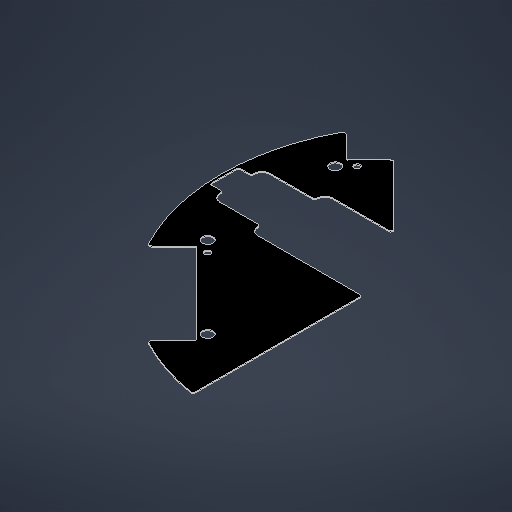
# Autodesk Inventor part: Cover Left
Saved by Autodesk Inventor 2026.1 (Build 301233020, 233B)
## iProperties
Created: 2026-06-25
Part Number: Cover Left
Material: Generic
Document SubType Name: Modeling
Designer: Bahaa
Mass: 3.13379 g
Surface Area: 128.68 cm^2
Volume: 3.13379 cm^3
Density: 1 g/cm^3
Appearance: Black PLA
Author: Bahaa
Autodesk Inventor part; units mm, degrees
ref_plane "YZ Plane" through (0, 0, 0) normal (1, 0, 0) x (0, 1, 0)
ref_plane "XZ Plane" through (0, 0, 0) normal (0, 1, 0) x (-1, 0, 0)
ref_plane "Work Plane1" through (0, 0, 0) normal (0, 0, 1) x (1, 0, 0)
sketch "Sketch1" plane through (0, 0, 0) normal (0, 0, 1) x (1, 0, 0)
  line L0 (-6.390879, 14.118801) -> (-6.390879, 24.738784)
  arc A0 (-4.409747, 26.159527) -> (-6.390879, 24.738784) centre (-4.890879, 24.738784) ccw
  arc A1 (11.10009, 19.508657) -> (-4.409747, 26.159527) centre (-38.890879, -75.660419) ccw
  arc A2 (11.463202, 17.120056) -> (11.10009, 19.508657) centre (10.402541, 18.180716) ccw
  line L1 (11.463202, 17.120056) -> (0.353553, 6.010408)
  arc A3 (-0.353553, 6.010408) -> (0.353553, 6.010408) centre (0, 6.363961) ccw
  line L2 (-0.353553, 6.010408) -> (-4.926413, 10.583267)
  arc A4 (-6.390879, 14.118801) -> (-4.926413, 10.583267) centre (-1.390879, 14.118801) ccw
  arc A5 (-78.135299, 6.01042) -> (-77.428193, 6.01042) centre (-77.781746, 6.363974) ccw
  line L3 (-78.135299, 6.01042) -> (-89.244944, 17.120065)
  arc A6 (-88.881832, 19.508666) -> (-89.244944, 17.120065) centre (-88.184283, 18.180725) ccw
  arc A7 (-73.372011, 26.159527) -> (-88.881832, 19.508666) centre (-38.890879, -75.660419) ccw
  arc A8 (-71.390879, 24.738784) -> (-73.372011, 26.159527) centre (-72.890879, 24.738784) ccw
  line L4 (-71.390879, 24.738784) -> (-71.390879, 14.118801)
  arc A9 (-72.855345, 10.583267) -> (-71.390879, 14.118801) centre (-76.390879, 14.118801) ccw
  line L5 (-72.855345, 10.583267) -> (-77.428193, 6.01042)
  circle A10 centre (-1.978787, -172.354511) radius 2.85
  circle A11 centre (36.76954, -114.551299) radius 1.6
  circle A12 centre (-114.551311, -114.551286) radius 1.6
  circle A13 centre (-114.551299, -36.76954) radius 1.6
  circle A14 centre (36.769553, -36.769553) radius 1.6
  circle A15 centre (-77.781759, -151.320838) radius 2.85
  circle A16 centre (-0.000013, -151.320851) radius 2.85
  circle A17 centre (42.426394, -108.894444) radius 2.85
  circle A18 centre (42.426394, -42.426394) radius 2.85
  circle A19 centre (-120.208153, -42.426394) radius 2.85
  circle A20 centre (-120.208153, -108.894444) radius 2.85
  arc A21 (-134.059964, -125.651371) -> (-131.671363, -126.014483) centre (-132.732023, -124.953823) ccw
  arc A22 (-134.059955, -25.66945) -> (-134.059964, -125.651371) centre (-38.890879, -75.660419) ccw
  arc A23 (-131.671354, -25.306338) -> (-134.059955, -25.66945) centre (-132.732015, -26.366998) ccw
  line L6 (-131.671354, -25.306338) -> (-120.561706, -36.415986)
  arc A24 (-120.561706, -36.415986) -> (-119.854599, -36.415986) centre (-120.208153, -36.062433) ccw
  line L7 (-119.854599, -36.415986) -> (-83.4386, 0.000013)
  line L8 (-83.4386, 0.000013) -> (-80.903066, -2.535521)
  arc A25 (-81.106225, -2.960902) -> (-80.903066, -2.535521) centre (-81.079843, -2.712298) ccw
  arc A26 (-81.106225, -2.960902) -> (-82.731493, -3.535521) centre (-81.31728, -4.949735) ccw
  line L9 (-82.731493, -3.535521) -> (-111.015777, -31.819805)
  arc A27 (-111.015777, -31.819805) -> (-111.015777, -34.648232) centre (-109.601564, -33.234019) ccw
  line L10 (-111.015777, -34.648232) -> (-110.308671, -35.355339)
  arc A28 (-110.308671, -38.183766) -> (-110.308671, -35.355339) centre (-111.722884, -36.769553) ccw
  line L11 (-110.308671, -38.183766) -> (-118.793939, -46.669035)
  arc A29 (-121.622366, -46.669035) -> (-118.793939, -46.669035) centre (-120.208153, -45.254821) ccw
  line L12 (-121.622366, -46.669035) -> (-128.634815, -39.656586)
  arc A30 (-128.634815, -39.656586) -> (-131.91894, -40.361269) centre (-130.049029, -41.0708) ccw
  arc A31 (-131.91894, -40.361269) -> (-138.034364, -67.24499) centre (-38.890879, -75.660419) ccw
  arc A32 (-139.030781, -68.160413) -> (-138.034364, -67.24499) centre (-139.030781, -67.160413) ccw
  line L13 (-139.030781, -68.160413) -> (-143.890873, -68.160413)
  arc A33 (-143.890873, -68.160413) -> (-144.890873, -69.160413) centre (-143.890873, -69.160413) ccw
  line L14 (-144.890873, -69.160413) -> (-144.890873, -82.160413)
  arc A34 (-144.890873, -82.160413) -> (-143.890873, -83.160413) centre (-143.890873, -82.160413) ccw
  line L15 (-143.890873, -83.160413) -> (-139.030782, -83.160413)
  arc A35 (-138.034365, -84.075836) -> (-139.030782, -83.160413) centre (-139.030782, -84.160413) ccw
  arc A36 (-138.034365, -84.075836) -> (-131.918947, -110.959551) centre (-38.890879, -75.660419) ccw
  arc A37 (-131.918947, -110.959551) -> (-128.634822, -111.664234) centre (-130.049036, -110.25002) ccw
  line L16 (-128.634822, -111.664234) -> (-121.622379, -104.651791)
  arc A38 (-118.793952, -104.651791) -> (-121.622379, -104.651791) centre (-120.208166, -106.066004) ccw
  line L17 (-118.793952, -104.651791) -> (-110.308671, -113.137072)
  arc A39 (-110.308671, -115.965499) -> (-110.308671, -113.137072) centre (-111.722884, -114.551286) ccw
  line L18 (-110.308671, -115.965499) -> (-111.015777, -116.672606)
  arc A40 (-111.015777, -116.672606) -> (-111.015777, -119.501033) centre (-109.601564, -118.08682) ccw
  line L19 (-111.015777, -119.501033) -> (-82.731493, -147.785317)
  arc A41 (-82.731493, -147.785317) -> (-79.903066, -147.785317) centre (-81.31728, -146.371104) ccw
  line L20 (-79.903066, -147.785317) -> (-79.195959, -147.07821)
  arc A42 (-76.367532, -147.07821) -> (-79.195959, -147.07821) centre (-77.781746, -148.492424) ccw
  line L21 (-76.367532, -147.07821) -> (-67.882264, -155.563479)
  arc A43 (-67.882264, -158.391906) -> (-67.882264, -155.563479) centre (-69.296477, -156.977693) ccw
  line L22 (-67.882264, -158.391906) -> (-74.894713, -165.404355)
  arc A44 (-74.894713, -165.404355) -> (-74.19003, -168.688479) centre (-73.480499, -166.818569) ccw
  arc A45 (-74.19003, -168.688479) -> (-56.419377, -173.60429) centre (-38.890879, -75.660419) ccw
  arc A46 (-56.419377, -173.60429) -> (-52.890879, -170.651208) centre (-55.890879, -170.651208) ccw
  line L23 (-52.890879, -170.651208) -> (-52.890879, -107.660419)
  arc A47 (-49.890879, -104.660419) -> (-52.890879, -107.660419) centre (-49.890879, -107.660419) ccw
  line L24 (-49.890879, -104.660419) -> (-27.890879, -104.660419)
  arc A48 (-24.890879, -107.660419) -> (-27.890879, -104.660419) centre (-27.890879, -107.660419) ccw
  line L25 (-24.890879, -107.660419) -> (-24.890879, -170.651208)
  arc A49 (-24.890879, -170.651208) -> (-21.362382, -173.60429) centre (-21.890879, -170.651208) ccw
  arc A50 (-21.362382, -173.60429) -> (-3.591748, -168.688487) centre (-38.890879, -75.660419) ccw
  arc A51 (-3.591748, -168.688487) -> (-2.887065, -165.404362) centre (-4.301278, -166.818576) ccw
  line L26 (-2.887065, -165.404362) -> (-9.899508, -158.391919)
  arc A52 (-9.899508, -155.563492) -> (-9.899508, -158.391919) centre (-8.485294, -156.977705) ccw
  line L27 (-9.899508, -155.563492) -> (-1.414226, -147.07821)
  arc A53 (1.414201, -147.07821) -> (-1.414226, -147.07821) centre (-0.000013, -148.492424) ccw
  line L28 (1.414201, -147.07821) -> (2.121308, -147.785317)
  arc A54 (2.121308, -147.785317) -> (4.949735, -147.785317) centre (3.535521, -146.371104) ccw
  line L29 (4.949735, -147.785317) -> (33.234019, -119.501033)
  arc A55 (33.234019, -119.501033) -> (33.234019, -116.672606) centre (31.819805, -118.08682) ccw
  line L30 (33.234019, -116.672606) -> (32.526912, -115.965499)
  arc A56 (32.526912, -113.137072) -> (32.526912, -115.965499) centre (33.941125, -114.551286) ccw
  line L31 (32.526912, -113.137072) -> (41.012181, -104.651804)
  arc A57 (43.840608, -104.651804) -> (41.012181, -104.651804) centre (42.426394, -106.066017) ccw
  line L32 (43.840608, -104.651804) -> (50.853057, -111.664252)
  arc A58 (50.853057, -111.664252) -> (54.137181, -110.95957) centre (52.26727, -110.250039) ccw
  arc A59 (54.137181, -110.95957) -> (54.137188, -40.361288) centre (-38.890879, -75.660419) ccw
  arc A60 (54.137188, -40.361288) -> (50.853064, -39.656604) centre (52.267277, -41.070818) ccw
  line L33 (50.853064, -39.656604) -> (43.84062, -46.669048)
  arc A61 (41.012193, -46.669048) -> (43.84062, -46.669048) centre (42.426407, -45.254834) ccw
  line L34 (41.012193, -46.669048) -> (32.526912, -38.183766)
  arc A62 (32.526912, -35.355339) -> (32.526912, -38.183766) centre (33.941125, -36.769553) ccw
  line L35 (32.526912, -35.355339) -> (33.234019, -34.648232)
  arc A63 (33.234019, -34.648232) -> (33.234019, -31.819805) centre (31.819805, -33.234019) ccw
  line L36 (33.234019, -31.819805) -> (4.949735, -3.535521)
  arc A64 (4.949735, -3.535521) -> (3.324466, -2.960902) centre (3.535521, -4.949735) ccw
  arc A65 (3.121308, -2.535521) -> (3.324466, -2.960902) centre (3.298084, -2.712298) ccw
  line L37 (3.121308, -2.535521) -> (5.656841, 0.000013)
  line L38 (5.656841, 0.000013) -> (42.072853, -36.415999)
  arc A66 (42.072853, -36.415999) -> (42.77996, -36.415999) centre (42.426407, -36.062446) ccw
  line L39 (42.77996, -36.415999) -> (53.889605, -25.306355)
  arc A67 (56.278205, -25.669467) -> (53.889605, -25.306355) centre (54.950265, -26.367015) ccw
  arc A68 (56.278197, -125.651388) -> (56.278205, -25.669467) centre (-38.890879, -75.660419) ccw
  arc A69 (53.889596, -126.0145) -> (56.278197, -125.651388) centre (54.950256, -124.95384) ccw
  line L40 (53.889596, -126.0145) -> (42.779948, -114.904852)
  arc A70 (42.779948, -114.904852) -> (42.072841, -114.904852) centre (42.426394, -115.258405) ccw
  line L41 (42.072841, -114.904852) -> (0.353541, -156.624152)
  arc A71 (0.353541, -156.624152) -> (0.353541, -157.331259) centre (0.707094, -156.977705) ccw
  line L42 (0.353541, -157.331259) -> (11.463185, -168.440903)
  arc A72 (11.100073, -170.829504) -> (11.463185, -168.440903) centre (10.402525, -169.501563) ccw
  arc A73 (-25.644434, -182.341166) -> (11.100073, -170.829504) centre (-38.890879, -75.660419) ccw
  arc A74 (-27.890879, -180.356408) -> (-25.644434, -182.341166) centre (-25.890879, -180.356408) ccw
  line L43 (-27.890879, -180.356408) -> (-27.890879, -108.660419)
  arc A75 (-27.890879, -108.660419) -> (-28.890879, -107.660419) centre (-28.890879, -108.660419) ccw
  line L44 (-28.890879, -107.660419) -> (-48.890879, -107.660419)
  arc A76 (-48.890879, -107.660419) -> (-49.890879, -108.660419) centre (-48.890879, -108.660419) ccw
  line L45 (-49.890879, -108.660419) -> (-49.890879, -180.356408)
  arc A77 (-52.137325, -182.341166) -> (-49.890879, -180.356408) centre (-51.890879, -180.356408) ccw
  arc A78 (-88.881849, -170.829495) -> (-52.137325, -182.341166) centre (-38.890879, -75.660419) ccw
  arc A79 (-89.24496, -168.440894) -> (-88.881849, -170.829495) centre (-88.1843, -169.501554) ccw
  line L46 (-89.24496, -168.440894) -> (-78.135312, -157.331246)
  arc A80 (-78.135312, -157.331246) -> (-78.135312, -156.624139) centre (-78.488865, -156.977693) ccw
  line L47 (-78.135312, -156.624139) -> (-119.854612, -114.904839)
  arc A81 (-119.854612, -114.904839) -> (-120.561719, -114.904839) centre (-120.208166, -115.258393) ccw
  line L48 (-120.561719, -114.904839) -> (-131.671363, -126.014483)
  circle A82 centre (-38.890886, -63.660413) radius 1.35
  circle A83 centre (-38.890886, -87.660413) radius 1.35
  arc A84 (-134.140886, -64.660413) -> (-136.140886, -66.660413) centre (-134.140886, -66.660413) ccw
  line L49 (-136.140886, -84.660413) -> (-136.140886, -66.660413)
  arc A85 (-136.140886, -84.660413) -> (-134.140886, -86.660413) centre (-134.140886, -84.660413) ccw
  line L50 (-113.140886, -86.660413) -> (-134.140886, -86.660413)
  arc A86 (-111.140886, -88.660413) -> (-113.140886, -86.660413) centre (-113.140886, -88.660413) ccw
  line L51 (-111.140886, -89.910413) -> (-111.140886, -88.660413)
  arc A87 (-111.140886, -89.910413) -> (-109.140886, -91.910413) centre (-109.140886, -89.910413) ccw
  line L52 (-3.890886, -91.910413) -> (-109.140886, -91.910413)
  arc A88 (-1.894796, -93.785413) -> (-3.890886, -91.910413) centre (-3.890886, -93.910413) ccw
  arc A89 (-1.894796, -93.785413) -> (0.101294, -95.660413) centre (0.101294, -93.660413) ccw
  line L53 (45.116934, -95.660413) -> (0.101294, -95.660413)
  arc A90 (45.116934, -95.660413) -> (47.113024, -93.785413) centre (45.116934, -93.660413) ccw
  arc A91 (49.109114, -91.910413) -> (47.113024, -93.785413) centre (49.109114, -93.910413) ccw
  line L54 (55.109114, -91.910413) -> (49.109114, -91.910413)
  arc A92 (55.109114, -91.910413) -> (57.109114, -89.910413) centre (55.109114, -89.910413) ccw
  line L55 (57.109114, -57.660413) -> (57.109114, -89.910413)
  arc A93 (57.109114, -57.660413) -> (55.109114, -55.660413) centre (55.109114, -57.660413) ccw
  line L56 (0.109114, -55.660413) -> (55.109114, -55.660413)
  arc A94 (0.109114, -55.660413) -> (-1.886976, -57.535413) centre (0.109114, -57.660413) ccw
  arc A95 (-3.883066, -59.410413) -> (-1.886976, -57.535413) centre (-3.883066, -57.410413) ccw
  line L57 (-106.640886, -59.410413) -> (-3.883066, -59.410413)
  arc A96 (-106.640886, -59.410413) -> (-108.640886, -61.410413) centre (-106.640886, -61.410413) ccw
  line L58 (-108.640886, -62.660413) -> (-108.640886, -61.410413)
  arc A97 (-110.640886, -64.660413) -> (-108.640886, -62.660413) centre (-110.640886, -62.660413) ccw
  line L59 (-134.140886, -64.660413) -> (-110.640886, -64.660413)
  line L60 (-104.298257, -25.102278) -> (-95.812976, -33.587559)
  line L61 (-95.812976, -33.587559) -> (-69.990122, -59.410413)
  line L62 (-38.890879, -91.910426) -> (-38.890879, -59.410413) construction
  line L63 (58.359127, -75.660426) -> (-136.140886, -75.660413) construction
  arc A98 (-3.883066, -57.410413) -> (-3.883066, -57.410413) centre (-3.883066, -57.410413) ccw
  arc A99 (0.109114, -53.660413) -> (-3.883066, -57.410413) centre (0.109114, -57.660413) ccw
  line L64 (0.109114, -53.660413) -> (55.109114, -53.660413)
  arc A100 (59.109114, -57.660413) -> (55.109114, -53.660413) centre (55.109114, -57.660413) ccw
  line L65 (59.109114, -57.660413) -> (59.109114, -89.910413)
  arc A101 (55.109114, -93.910413) -> (59.109114, -89.910413) centre (55.109114, -89.910413) ccw
  line L66 (55.109114, -93.910413) -> (49.109114, -93.910413)
  arc A102 (49.109114, -93.910413) -> (49.109114, -93.910413) centre (49.109114, -93.910413) ccw
  arc A103 (45.116934, -97.660413) -> (49.109114, -93.910413) centre (45.116934, -93.660413) ccw
  line L67 (45.116934, -97.660413) -> (0.101294, -97.660413)
  arc A104 (-3.890886, -93.910413) -> (0.101294, -97.660413) centre (0.101294, -93.660413) ccw
  arc A105 (-3.890886, -93.910413) -> (-3.890886, -93.910413) centre (-3.890886, -93.910413) ccw
  line L68 (-3.890886, -93.910413) -> (-109.140886, -93.910413)
  arc A106 (-113.140886, -89.910413) -> (-109.140886, -93.910413) centre (-109.140886, -89.910413) ccw
  line L69 (-113.140886, -89.910413) -> (-113.140886, -88.660413)
  arc A107 (-113.140886, -88.660413) -> (-113.140886, -88.660413) centre (-113.140886, -88.660413) ccw
  line L70 (-113.140886, -88.660413) -> (-134.140886, -88.660413)
  arc A108 (-138.140886, -84.660413) -> (-134.140886, -88.660413) centre (-134.140886, -84.660413) ccw
  line L71 (-138.140886, -84.660413) -> (-138.140886, -66.660413)
  arc A109 (-134.140886, -62.660413) -> (-138.140886, -66.660413) centre (-134.140886, -66.660413) ccw
  line L72 (-134.140886, -62.660413) -> (-110.640886, -62.660413)
  arc A110 (-110.640886, -62.660413) -> (-110.640886, -62.660413) centre (-110.640886, -62.660413) ccw
  line L73 (-110.640886, -62.660413) -> (-110.640886, -61.410413)
  arc A111 (-106.640886, -57.410413) -> (-110.640886, -61.410413) centre (-106.640886, -61.410413) ccw
  line L74 (-106.640886, -57.410413) -> (-3.883066, -57.410413)
  line L75 (-105.71247, -26.516492) -> (-97.227189, -35.001773)
  line L76 (-97.227189, -35.001773) -> (-71.404336, -60.824626)
  line L77 (-38.890879, -151.320851) -> (-38.890879, 0.000013)
  line L78 (-27.890879, -102.660419) -> (-49.890879, -102.660419)
  arc A112 (-49.890879, -102.660419) -> (-54.890879, -107.660419) centre (-49.890879, -107.660419) ccw
  line L79 (-54.890879, -107.660419) -> (-54.890879, -170.651208)
  arc A113 (-56.067045, -171.635569) -> (-54.890879, -170.651208) centre (-55.890879, -170.651208) ccw
  arc A114 (-73.480499, -166.818569) -> (-56.067045, -171.635569) centre (-38.890879, -75.660419) ccw
  line L80 (-73.480499, -166.818569) -> (-66.46805, -159.80612)
  arc A115 (-66.46805, -159.80612) -> (-66.46805, -154.149266) centre (-69.296477, -156.977693) ccw
  line L81 (-66.46805, -154.149266) -> (-74.953319, -145.663997)
  arc A116 (-74.953319, -145.663997) -> (-80.610173, -145.663997) centre (-77.781746, -148.492424) ccw
  line L82 (-80.610173, -145.663997) -> (-81.31728, -146.371104)
  line L83 (-81.31728, -146.371104) -> (-109.601564, -118.08682)
  line L84 (-109.601564, -118.08682) -> (-108.894457, -117.379713)
  arc A117 (-108.894457, -117.379713) -> (-108.894457, -111.722859) centre (-111.722884, -114.551286) ccw
  line L85 (-108.894457, -111.722859) -> (-117.379738, -103.237577)
  arc A118 (-117.379738, -103.237577) -> (-123.036593, -103.237577) centre (-120.208166, -106.066004) ccw
  line L86 (-123.036593, -103.237577) -> (-130.049036, -110.25002)
  arc A119 (-136.041531, -83.906682) -> (-130.049036, -110.25002) centre (-38.890879, -75.660419) ccw
  arc A120 (-136.041531, -83.906682) -> (-139.030782, -81.160413) centre (-139.030782, -84.160413) ccw
  line L87 (-139.030782, -81.160413) -> (-142.890873, -81.160413)
  line L88 (-142.890873, -81.160413) -> (-142.890873, -70.160413)
  line L89 (-142.890873, -70.160413) -> (-139.030781, -70.160413)
  arc A121 (-139.030781, -70.160413) -> (-136.04153, -67.414144) centre (-139.030781, -67.160413) ccw
  arc A122 (-130.049029, -41.0708) -> (-136.04153, -67.414144) centre (-38.890879, -75.660419) ccw
  line L90 (-130.049029, -41.0708) -> (-123.03658, -48.083248)
  arc A123 (-123.03658, -48.083248) -> (-117.379726, -48.083248) centre (-120.208153, -45.254821) ccw
  line L91 (-117.379726, -48.083248) -> (-108.894457, -39.59798)
  arc A124 (-108.894457, -39.59798) -> (-108.894457, -33.941125) centre (-111.722884, -36.769553) ccw
  line L92 (-108.894457, -33.941125) -> (-109.601564, -33.234019)
  line L93 (-109.601564, -33.234019) -> (-81.31728, -4.949735)
  arc A125 (-81.31728, -4.949735) -> (-79.488853, -1.121308) centre (-81.079843, -2.712298) ccw
  line L94 (-79.488853, -1.121308) -> (-83.4386, 2.82844)
  line L95 (-83.4386, 2.82844) -> (-120.208153, -33.941113)
  line L96 (-120.208153, -33.941113) -> (-130.257141, -23.892125)
  arc A126 (-130.257141, -23.892125) -> (-135.830543, -24.739385) centre (-132.732015, -26.366998) ccw
  arc A127 (-135.830543, -24.739385) -> (-135.830552, -126.581436) centre (-38.890879, -75.660419) ccw
  arc A128 (-135.830552, -126.581436) -> (-130.25715, -127.428697) centre (-132.732023, -124.953823) ccw
  line L97 (-130.25715, -127.428697) -> (-120.208166, -117.379713)
  line L98 (-120.208166, -117.379713) -> (-80.610186, -156.977693)
  line L99 (-80.610186, -156.977693) -> (-90.659174, -167.026681)
  arc A129 (-90.659174, -167.026681) -> (-89.811913, -172.600083) centre (-88.1843, -169.501554) ccw
  arc A130 (-89.811913, -172.600083) -> (-52.38377, -184.325924) centre (-38.890879, -75.660419) ccw
  arc A131 (-52.38377, -184.325924) -> (-47.890879, -180.356408) centre (-51.890879, -180.356408) ccw
  line L100 (-47.890879, -180.356408) -> (-47.890879, -109.660419)
  line L101 (-47.890879, -109.660419) -> (-29.890879, -109.660419)
  line L102 (-29.890879, -109.660419) -> (-29.890879, -180.356408)
  arc A132 (-29.890879, -180.356408) -> (-25.397988, -184.325924) centre (-25.890879, -180.356408) ccw
  arc A133 (-25.397988, -184.325924) -> (12.030137, -172.600092) centre (-38.890879, -75.660419) ccw
  arc A134 (12.030137, -172.600092) -> (12.877398, -167.02669) centre (10.402525, -169.501563) ccw
  line L103 (12.877398, -167.02669) -> (2.828414, -156.977705)
  line L104 (2.828414, -156.977705) -> (42.426394, -117.379726)
  line L105 (42.426394, -117.379726) -> (52.475382, -127.428714)
  arc A135 (52.475382, -127.428714) -> (58.048784, -126.581453) centre (54.950256, -124.95384) ccw
  arc A136 (58.048784, -126.581453) -> (58.048793, -24.739403) centre (-38.890879, -75.660419) ccw
  arc A137 (58.048793, -24.739403) -> (52.475391, -23.892141) centre (54.950265, -26.367015) ccw
  line L106 (52.475391, -23.892141) -> (42.426407, -33.941125)
  line L107 (42.426407, -33.941125) -> (5.656841, 2.82844)
  line L108 (5.656841, 2.82844) -> (1.707094, -1.121308)
  arc A138 (1.707094, -1.121308) -> (3.535521, -4.949735) centre (3.298084, -2.712298) ccw
  line L109 (3.535521, -4.949735) -> (31.819805, -33.234019)
  line L110 (31.819805, -33.234019) -> (31.112698, -33.941125)
  arc A139 (31.112698, -33.941125) -> (31.112698, -39.59798) centre (33.941125, -36.769553) ccw
  line L111 (31.112698, -39.59798) -> (39.59798, -48.083261)
  arc A140 (39.59798, -48.083261) -> (45.254834, -48.083261) centre (42.426407, -45.254834) ccw
  line L112 (45.254834, -48.083261) -> (52.267277, -41.070818)
  arc A141 (52.26727, -110.250039) -> (52.267277, -41.070818) centre (-38.890879, -75.660419) ccw
  line L113 (52.26727, -110.250039) -> (45.254821, -103.23759)
  arc A142 (45.254821, -103.23759) -> (39.597967, -103.23759) centre (42.426394, -106.066017) ccw
  line L114 (39.597967, -103.23759) -> (31.112698, -111.722859)
  arc A143 (31.112698, -111.722859) -> (31.112698, -117.379713) centre (33.941125, -114.551286) ccw
  line L115 (31.112698, -117.379713) -> (31.819805, -118.08682)
  line L116 (31.819805, -118.08682) -> (3.535521, -146.371104)
  line L117 (3.535521, -146.371104) -> (2.828414, -145.663997)
  arc A144 (2.828414, -145.663997) -> (-2.82844, -145.663997) centre (-0.000013, -148.492424) ccw
  line L118 (-2.82844, -145.663997) -> (-11.313721, -154.149278)
  arc A145 (-11.313721, -154.149278) -> (-11.313721, -159.806133) centre (-8.485294, -156.977705) ccw
  line L119 (-11.313721, -159.806133) -> (-4.301278, -166.818576)
  arc A146 (-21.714714, -171.635569) -> (-4.301278, -166.818576) centre (-38.890879, -75.660419) ccw
  arc A147 (-22.890879, -170.651208) -> (-21.714714, -171.635569) centre (-21.890879, -170.651208) ccw
  line L120 (-22.890879, -170.651208) -> (-22.890879, -107.660419)
  arc A148 (-22.890879, -107.660419) -> (-27.890879, -102.660419) centre (-27.890879, -107.660419) ccw
  line L121 (-105.71247, -26.516492) -> (-109.248001, -22.980961)
  line L122 (-54.890879, -107.660419) -> (-54.890879, -93.910413)
  line L123 (-54.890879, -170.651208) -> (-54.890879, -183.985162)
  line L124 (-86.140886, -68.682856) -> (-138.140886, -68.682856)
  line L125 (-136.140886, -68.682856) -> (-136.140886, -82.637973)
  line L126 (-138.140886, -82.637973) -> (-86.140886, -82.637973)
  line L127 (-86.140886, -82.637973) -> (-86.140886, -68.682856)
  line L128 (-86.140886, -68.682856) -> (-136.140886, -82.637973) construction
  line L129 (-136.140886, -68.682856) -> (-86.140886, -82.637973) construction
  point P0 (0, 0)
  point P1 (-74.818549, -57.410413)
  point P2 (-38.890879, -109.660419)
  point P3 (-38.890879, -93.910413)
  point P4 (-138.140886, -83.70425)
  point P5 (-138.140886, -67.616578)
  point P6 (-135.554712, -88.402216)
  point P7 (-105.712467, -26.516495)
  point P8 (-137.830542, -65.115603)
  point P9 (-52.890879, -184.261754)
  point P10 (-38.890879, -104.660419)
  point P11 (-38.890879, -57.410413)
  point P12 (56.972487, -93.449882)
  point P13 (56.124921, -53.791545)
  point P14 (-138.140886, -81.295437)
  point P15 (-138.140886, -70.025389)
  point P16 (-104.298254, -27.930708)
  point P17 (-107.833787, -24.395175)
  point P18 (-135.554711, -62.918609)
  point P19 (-38.890879, -102.660419)
  point P20 (-38.890879, -107.660419)
  point P21 (58.581192, -55.674292)
  point P22 (59.109114, -58.448468)
  point P23 (-137.830544, -86.205218)
  point P24 (-38.890879, -65.010413)
  point P25 (-38.890879, -62.310413)
  point P26 (-38.890879, -89.010413)
  point P27 (-38.890879, -86.310413)
  point P28 (-135.877526, -65.668405)
  point P29 (-136.140886, -67.965711)
  point P30 (56.696667, -56.443993)
  point P31 (57.109114, -58.623658)
  point P32 (-135.877528, -85.652418)
  point P33 (-136.140886, -83.355118)
  point P34 (-111.140886, -75.660414)
  point P35 (-136.140886, -75.660414)
  point P36 (-54.890879, -181.963053)
  dimension "d0" = 2
  dimension "d1" = 2
  dimension "d2" = 2
  dimension "d6" = 50
  constraints: 238 end point, 236 point on circle, 133 centre point, 11 point on line, 10 coincident with centre, 8 vertical, 7 midpoint, 5 horizontal, 4 perpendicular, 2 parallel, 429 other
  measures "d0" distance between parallel lines of L57 L74
  measures "d1" distance between parallel lines of L60 L75
  measures "d2" distance between parallel lines of L24 L78
  measures "d6" distance from line of point (-136.141, -75.66) L127
sketch "Sketch1 outline for Extrusion1" plane through (0, 0, 0) normal (0, 0, 1) x (1, 0, 0)
  line L0 (-134.140886, -62.660413) -> (-110.640886, -62.660413)
  arc A0 (-138.140886, -66.660413) -> (-134.140886, -62.660413) centre (-134.140886, -66.660413) cw
  line L1 (-110.640886, -62.660413) -> (-110.640886, -61.410413)
  line L2 (-138.140886, -67.616578) -> (-138.140886, -66.660413)
  arc A1 (-110.640886, -61.410413) -> (-106.640886, -57.410413) centre (-106.640886, -61.410413) cw
  arc A2 (-139.030781, -68.160413) -> (-138.140886, -67.616578) centre (-139.030781, -67.160413) ccw
  line L3 (-106.640886, -57.410413) -> (-74.818549, -57.410413)
  line L4 (-143.890873, -68.160413) -> (-139.030781, -68.160413)
  line L5 (-74.818549, -57.410413) -> (-97.227189, -35.001773)
  arc A3 (-144.890873, -69.160413) -> (-143.890873, -68.160413) centre (-143.890873, -69.160413) cw
  line L6 (-97.227189, -35.001773) -> (-105.71247, -26.516492)
  line L7 (-144.890873, -82.160413) -> (-144.890873, -69.160413)
  line L8 (-105.71247, -26.516492) -> (-107.833787, -24.395175)
  arc A4 (-143.890873, -83.160413) -> (-144.890873, -82.160413) centre (-143.890873, -82.160413) cw
  line L9 (-107.833787, -24.395175) -> (-119.854599, -36.415986)
  line L10 (-139.030782, -83.160413) -> (-143.890873, -83.160413)
  arc A5 (-119.854599, -36.415986) -> (-120.561706, -36.415986) centre (-120.208153, -36.062433) cw
  arc A6 (-138.140886, -83.70425) -> (-139.030782, -83.160413) centre (-139.030782, -84.160413) ccw
  line L11 (-120.561706, -36.415986) -> (-131.671354, -25.306338)
  line L12 (-138.140886, -84.660413) -> (-138.140886, -83.70425)
  arc A7 (-131.671354, -25.306338) -> (-134.059955, -25.66945) centre (-132.732015, -26.366998) ccw
  arc A8 (-134.140886, -88.660413) -> (-138.140886, -84.660413) centre (-134.140886, -84.660413) cw
  arc A9 (-134.059955, -25.66945) -> (-134.059964, -125.651371) centre (-38.890879, -75.660419) ccw
  line L13 (-113.140886, -88.660413) -> (-134.140886, -88.660413)
  arc A10 (-134.059964, -125.651371) -> (-131.671363, -126.014483) centre (-132.732023, -124.953823) ccw
  line L14 (-113.140886, -89.910413) -> (-113.140886, -88.660413)
  line L15 (-131.671363, -126.014483) -> (-120.561719, -114.904839)
  arc A11 (-109.140886, -93.910413) -> (-113.140886, -89.910413) centre (-109.140886, -89.910413) cw
  arc A12 (-120.561719, -114.904839) -> (-119.854612, -114.904839) centre (-120.208166, -115.258393) cw
  line L16 (-54.890879, -93.910413) -> (-109.140886, -93.910413)
  line L17 (-119.854612, -114.904839) -> (-78.135312, -156.624139)
  line L18 (-54.890879, -107.660419) -> (-54.890879, -93.910413)
  arc A13 (-78.135312, -156.624139) -> (-78.135312, -157.331246) centre (-78.488865, -156.977693) cw
  line L19 (-54.890879, -170.651208) -> (-54.890879, -107.660419)
  line L20 (-78.135312, -157.331246) -> (-89.24496, -168.440894)
  line L21 (-54.890879, -181.963053) -> (-54.890879, -170.651208)
  arc A14 (-89.24496, -168.440894) -> (-88.881849, -170.829495) centre (-88.1843, -169.501554) ccw
  arc A15 (-88.881849, -170.829495) -> (-54.890879, -181.963053) centre (-38.890879, -75.660419) ccw
  circle A16 centre (-114.551311, -114.551286) radius 1.6
  circle A17 centre (-120.208153, -108.894444) radius 2.85
  circle A18 centre (-77.781759, -151.320838) radius 2.85
  circle A19 centre (-120.208153, -42.426394) radius 2.85
  circle A20 centre (-114.551299, -36.76954) radius 1.6
extrude "Extrusion1" add sketch "Sketch1 outline for Extrusion1" along normal blind 0.5
fillet "Fillet1" radius 1 6 edges at (-74.8185, -57.4104, 0.25) (-110.6409, -62.6604, 0.25) (-113.1409, -88.6604, 0.25) (-54.8909, -93.9104, 0.25) (-54.8909, -181.9631, 0.25) (-107.8338, -24.3952, 0.25)
body "Solid1"
